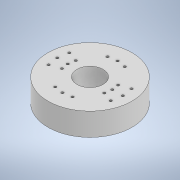
# Autodesk Inventor part: engine_connector_sleeve
Saved by Autodesk Inventor 2020.1 (Build 241239000, 239)
## iProperties
Created: 2022-02-06
Part Number: engine_connector_sleeve
Material: Generic
Document SubType Name: Modeling
Designer: OEM
Density: 1 g/cm^3
Appearance: Default
Author: OEM
Autodesk Inventor part; units mm, degrees
ref_plane "YZ Plane" through (0, 0, 0) normal (1, 0, 0) x (0, 1, 0)
ref_plane "XZ Plane" through (0, 0, 0) normal (0, 1, 0) x (-1, 0, 0)
ref_plane "XY Plane" through (0, 0, 0) normal (0, 0, 1) x (1, 0, 0)
sketch "Sketch1" plane through (0, 0, 0) normal (0, 1, 0) x (-1, 0, 0)
  circle A0 centre (0, 0) radius 12
  circle A1 centre (-0.0043, 0) radius 3.75
  circle A2 centre (-0.0043, 0) radius 6.375 construction
  circle A3 centre (-0.0043, 0) radius 9.375 construction
  circle A4 centre (-0.0043, 0) radius 7.875 construction
  circle A5 centre (0, -7.875) radius 0.35
  circle A6 centre (6.3707, 0) radius 0.35
  circle A7 centre (9.3707, 0) radius 0.35
  line L0 (16.292, 0) -> (-19, 0) construction
  line L1 (0, 21) -> (0, -27.3544) construction
  circle A8 centre (0, 7.875) radius 0.35
  circle A9 centre (-6.3707, 0) radius 0.35
  circle A10 centre (-9.3707, 0) radius 0.35
  line L2 (-0.0043, 0) -> (-8.4874, 8.4831) construction
  line L3 (-0.0043, 0) -> (11.9927, 0) construction
  circle A11 centre (-5.5728, 5.5685) radius 0.75
  circle A12 centre (5.5728, 5.5685) radius 0.75
  circle A13 centre (-5.5728, -5.5685) radius 0.75
  circle A14 centre (5.5728, -5.5685) radius 0.75
  circle A15 centre (-2.4685, 7.4795) radius 0.35
  circle A16 centre (2.4685, 7.4795) radius 0.35
  circle A17 centre (-2.4685, -7.4795) radius 0.35
  circle A18 centre (2.4685, -7.4795) radius 0.35
  circle A19 centre (6.057, 1.9752) radius 0.35
  circle A20 centre (8.8907, 2.9614) radius 0.35
  circle A21 centre (6.057, -1.9752) radius 0.35
  circle A22 centre (8.8907, -2.9614) radius 0.35
  circle A23 centre (-6.057, 1.9752) radius 0.35
  circle A24 centre (-8.8907, 2.9614) radius 0.35
  circle A25 centre (-8.8907, -2.9614) radius 0.35
  circle A26 centre (-6.057, -1.9752) radius 0.35
  dimension "d4" = 24
  dimension "d2" = 7.5
  dimension "d6" = 12.75
  dimension "d7" = 18.75
  dimension "d8" = 15.75
  dimension "d9" = 0.7
  dimension "d13" = 0.7
  dimension "d14" = 0.7
  dimension "d27" = 135
  dimension "d29" = 0.7
  dimension "d33" = 1.8
  dimension "d34" = 1.5
  dimension "d35" = 1.3
  dimension "d36" = 0.7
  dimension "d37" = 0.7
  dimension "d38" = 2.3
  constraints: 26 centre point, 15 symmetric about line, 8 end point, 8 point on circle, 6 point on line, 4 coincident, 2 horizontal, 1 equal length, 1 vertical, 18 other
  measures "d2" diameter of A1
  measures "d6" diameter of A2
  measures "d7" diameter of A3
  measures "d8" diameter of A4
  measures "d9" diameter of A5
  measures "d13" diameter of A6
  measures "d14" diameter of A7
  measures "d27" angle of L3 L2
  measures "d29" diameter of A15
  measures "d34" diameter of A11
  measures "d36" diameter of A19
  measures "d37" diameter of A20
extrude "Extrusion4" add sketch "Sketch1" along normal blind 6.5 contours A0 | A11 | A12 | A13 | A14
extrude "Extrusion5" add sketch "Sketch1" along normal blind 3.5 contours A5 | A6 | A7 | A8 | A9 | A10 | A15 | A16 | A17 | A18 | A19 | A20 | A21 | A22 | A23 | A24 | A25 | A26
extrude "Extrusion6" cut sketch "Sketch1" along normal blind 4 contours A11 | A12 | A13 | A14
equation "\"d13\" = d9"
equation "\"d14\" = d9"
equation "\"d29\" = d9"
equation "\"d36\" = d13"
equation "\"d37\" = d14"
body "Solid2"
